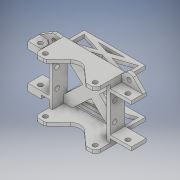
# Autodesk Inventor part: 14HM08 Chassis Flat Bottom
Saved by Autodesk Inventor 2019 (Build 230136000, 136)
## iProperties
Created: 2019-01-31
Part Number: 14HM08 Chassis Flat Bottom
Material: Generic
Document SubType Name: Modeling
Designer: Billy
Density: 1 g/cm^3
Appearance: Red
Author: Billy
Autodesk Inventor part; units mm, degrees
note: some values were not read from the file. Chosen so that the rebuilt part matches the saved one: sketch regions of "Extrusion3".
ref_plane "YZ Plane" through (0, 0, 0) normal (1, 0, 0) x (0, 1, 0)
ref_plane "XZ Plane" through (0, 0, 0) normal (0, 1, 0) x (-1, 0, 0)
sketch "Sketch1" plane through (0, 0, 0) normal (0, 1, 0) x (-1, 0, 0)
  circle A0 centre (21.95, 0) radius 2
  circle A1 centre (-21.95, 0) radius 2
  arc A2 (26.95, 0) -> (18.533144, 3.650355) centre (21.95, 0) ccw
  arc A3 (-18.533144, 3.650355) -> (-26.95, 0) centre (-21.95, 0) ccw
  arc A4 (-6.833713, -7.30071) -> (6.833713, -7.30071) centre (0, 0) ccw
  line L0 (6.833713, -7.30071) -> (18.533144, 3.650355)
  line L1 (-6.833713, -7.30071) -> (-18.533144, 3.650355)
  line L2 (-26.95, 0) -> (-26.95, -18.25)
  line L3 (-26.95, -18.25) -> (26.95, -18.25)
  line L4 (26.95, -18.25) -> (26.95, 0)
  constraints: 10 end point, 6 point on circle, 5 centre point, 4 tangent, 3 coincident, 1 parallel, 5 other
extrude "Extrusion1" add sketch "Sketch1" along normal blind 3
ref_plane "Work Plane1" through (0, 48, 0) normal (0, 1, 0) x (1, 0, 0)
sketch "Sketch2" plane through (0, 48, 0) normal (0, 1, 0) x (1, 0, 0)
  circle A0 centre (21.95, 0) radius 2
  circle A1 centre (-21.95, 0) radius 2
  line L0 (-18.533144, -3.650355) -> (-6.833713, 7.30071)
  arc A2 (6.833713, 7.30071) -> (-6.833713, 7.30071) centre (0, 0) ccw
  line L1 (6.833713, 7.30071) -> (18.533144, -3.650355)
  arc A3 (18.533144, -3.650355) -> (26.95, 0) centre (21.95, 0) ccw
  line L2 (26.95, 0) -> (26.95, 18.25)
  line L3 (26.95, 18.25) -> (-26.95, 18.25)
  line L4 (-26.95, 18.25) -> (-26.95, 0)
  arc A4 (-26.95, 0) -> (-18.533144, -3.650355) centre (-21.95, 0) ccw
extrude "Extrusion2" add sketch "Sketch2" along normal blind 3
sketch "Sketch3" plane through (26.95, 48, -18.25) normal (0, 0, -1) x (-1, 0, 0)
  line L0 (0, 0) -> (53.9, 0)
  line L1 (53.9, 0) -> (53.9, 3)
  line L2 (0, 3) -> (53.9, 3)
  line L3 (0, 0) -> (0, 3)
  line L4 (53.9, -48) -> (0, -48)
  line L5 (53.9, -48) -> (53.9, -45)
  line L6 (0, -45) -> (53.9, -45)
  line L7 (0, -48) -> (0, -45)
  circle A0 centre (-6.625, -46.63) radius 2
  circle A1 centre (-6.625, 1.63) radius 2
  circle A2 centre (59.415, -43.455) radius 2
  circle A3 centre (59.415, -1.545) radius 2
  arc A4 (58.987392, -48.436682) -> (59.415, -38.455) centre (59.415, -43.455) ccw
  arc A5 (-6.625, -41.63) -> (-3.688232, -50.676652) centre (-6.625, -46.63) ccw
  arc A6 (59.415, -6.545) -> (58.987392, 3.436682) centre (59.415, -1.545) ccw
  arc A7 (-3.688232, 5.676652) -> (-6.625, -3.37) centre (-6.625, 1.63) ccw
  line L8 (53.9, -48) -> (0, -48)
  line L9 (0, 3) -> (53.9, 3)
  line L10 (0, -48) -> (-3.688232, -50.676652)
  line L11 (-6.625, -41.63) -> (0, -41.63)
  line L12 (53.9, -48) -> (58.987392, -48.436682)
  line L13 (59.415, -38.455) -> (53.9, -38.455)
  line L14 (53.9, -45) -> (53.9, -48)
  line L15 (0, -48) -> (0, -45)
  line L16 (59.415, -6.545) -> (53.9, -6.545)
  line L17 (53.9, 3) -> (58.987392, 3.436682)
  line L18 (53.9, 3) -> (53.9, 0)
  line L19 (53.9, -6.545) -> (53.9, -38.455)
  line L20 (0, 3) -> (-3.688232, 5.676652)
  line L21 (-6.625, -3.37) -> (0, -3.37)
  line L22 (0, -41.63) -> (0, -3.37)
  line L23 (0, 0) -> (0, 3)
  point P0 (26.95, -48)
  constraints: 36 end point, 10 parallel, 10 perpendicular, 8 centre point, 8 point on circle, 6 tangent, 4 coincident, 2 horizontal, 2 vertical, 8 other
extrude "Extrusion3" add sketch "Sketch3" along normal blind 3
sketch "Sketch4" plane through (26.95, 0, 0) normal (1, 0, 0) x (0, 0, -1)
  line L0 (18.25, 3) -> (0, 3)
  line L1 (7.30071, 48) -> (10, 48)
  line L2 (18.25, 3) -> (8.25, 3)
  line L3 (8.25, 3) -> (8.25, 48)
  line L4 (8.25, 48) -> (18.25, 48)
  line L5 (18.25, 48) -> (18.25, 3)
  point P0 (0, 0)
  dimension "d34" = 10
  constraints: 8 end point, 2 parallel, 1 horizontal, 1 perpendicular, 1 point on line
  measures "d34" distance of L3.end L4.end
extrude "Extrusion4" add sketch "Sketch4" against normal blind 3
sketch "Sketch5" plane through (-26.95, 0, 0) normal (-1, 0, 0) x (0, 0, 1)
  line L0 (-8.25, 3) -> (-18.25, 3) projected
  line L1 (-8.25, 3) -> (-8.25, 48) projected
  line L2 (-18.25, 48) -> (-8.25, 48) projected
  line L3 (-18.25, 3) -> (-18.25, 48) projected
  point P0 (0, 0)
extrude "Extrusion5" add sketch "Sketch5" against normal blind 3
sketch "Sketch6" plane through (26.95, 48, -18.25) normal (0, 0, 1) x (1, 0, 0)
  line L0 (-50.9, -6.860357) -> (-50.9, -38.139643)
  line L1 (-10.302469, -45) -> (-43.597531, -45)
  line L2 (-3, -38.139643) -> (-3, -6.860357)
  line L3 (-10.302469, 0) -> (-43.597531, 0)
  line L4 (-50.9, -38.139643) -> (-34.252469, -22.5)
  line L5 (-26.95, -15.639643) -> (-10.302469, 0)
  line L6 (-10.302469, -45) -> (-26.95, -29.360357)
  line L7 (-34.252469, -22.5) -> (-50.9, -6.860357)
  line L8 (-3, -38.139643) -> (-19.647531, -22.5)
  line L9 (-26.95, -15.639643) -> (-43.597531, 0)
  line L10 (-43.597531, -45) -> (-26.95, -29.360357)
  line L11 (-19.647531, -22.5) -> (-3, -6.860357)
  point P0 (-26.95, -48)
  constraints: 24 end point
extrude "Extrusion6" cut sketch "Sketch6" against normal blind 3
sketch "Sketch8" plane through (26.95, 48, -21.25) normal (0, 0, -1) x (-1, 0, 0)
  line L0 (10.302469, -45) -> (26.95, -29.360357)
  line L1 (26.95, -29.360357) -> (43.597531, -45)
  line L2 (43.597531, -45) -> (10.302469, -45)
  line L3 (43.597531, 0) -> (26.95, -15.639643)
  line L4 (26.95, -15.639643) -> (10.302469, 0)
  line L5 (10.302469, 0) -> (43.597531, 0)
  line L6 (3, -6.860357) -> (19.647531, -22.5)
  line L7 (19.647531, -22.5) -> (3, -38.139643)
  line L8 (3, -38.139643) -> (3, -6.860357)
  line L9 (50.9, -38.139643) -> (34.252469, -22.5)
  line L10 (34.252469, -22.5) -> (50.9, -6.860357)
  line L11 (50.9, -6.860357) -> (50.9, -38.139643)
  circle A0 centre (59.415, -1.545) radius 2
  circle A1 centre (59.415, -43.455) radius 2
  circle A2 centre (-6.625, 1.63) radius 2
  circle A3 centre (-6.625, -46.63) radius 2
  line L12 (0, 3) -> (-3.688232, 5.676652)
  arc A4 (-3.688232, 5.676652) -> (-6.625, -3.37) centre (-6.625, 1.63) ccw
  arc A5 (-6.625, -41.63) -> (-3.688232, -50.676652) centre (-6.625, -46.63) ccw
  line L13 (-3.688232, -50.676652) -> (0, -48)
  line L14 (0, -48) -> (53.9, -48)
  line L15 (53.9, -48) -> (58.987392, -48.436682)
  arc A6 (58.987392, -48.436682) -> (59.415, -38.455) centre (59.415, -43.455) ccw
  line L16 (59.415, -38.455) -> (53.9, -38.455)
  line L17 (57.121975, -6.545) -> (59.415, -6.545)
  arc A7 (59.415, -6.545) -> (58.987392, 3.436682) centre (59.415, -1.545) ccw
  line L18 (58.987392, 3.436682) -> (53.9, 3)
  line L19 (53.9, 3) -> (0, 3)
  line L20 (53.9, -40.75) -> (0, -40.75)
  line L21 (53.9, -4.25) -> (0, -4.25)
  line L22 (0, -41.63) -> (0, -43.75)
  line L23 (0, -1.25) -> (0, -4.25)
  line L24 (0, -40.75) -> (0, -41.63)
  line L25 (63.620113, -43.75) -> (57.436876, -43.75)
  line L26 (53.9, -43.75) -> (0, -43.75)
  line L27 (63.620113, -1.25) -> (57.436876, -1.25)
  line L28 (53.9, -1.25) -> (0, -1.25)
  line L29 (53.9, -43.75) -> (53.9, -40.75)
  line L30 (53.9, -4.25) -> (53.9, -1.25)
  point P0 (26.95, -48)
  constraints: 62 end point, 8 centre point, 4 point on circle, 1 point on line, 18 other
extrude "Extrusion7" add sketch "Sketch8" along normal blind 18 contours L26 L22 L24 L20 L0 | L0 L20 L1 L26 | L1 L20 L29 L26 | L28 L30 L21 L3 | L3 L21 L4 L28 | L4 L21 L23 L28
sketch "Sketch9" plane through (-12.123642, 43.75, -21.25) normal (0, -1, 0) x (1, 0, 0)
  line L0 (24.247285, 0) -> (39.073642, 0)
  line L1 (24.247285, 0) -> (0, 0)
  line L2 (-14.826358, 0) -> (0, 0)
  line L3 (-14.826358, 0) -> (-14.826358, -18)
  line L4 (39.073642, -18) -> (-14.826358, -18)
  line L5 (39.073642, 0) -> (39.073642, -18)
  line L6 (-11.826358, -15) -> (-11.826358, -3)
  line L7 (0, -3) -> (24.247285, -3)
  line L8 (36.073642, -3) -> (36.073642, -15)
  line L9 (23.776294, -15) -> (0.470991, -15)
  line L10 (-8.512342, -18) -> (-14.192846, -19.897014)
  line L11 (38.440131, -19.897014) -> (32.759627, -18)
  line L12 (12.123642, -11.108577) -> (0.470991, -15)
  line L13 (23.776294, -15) -> (12.123642, -11.108577)
  line L14 (5.809627, -9) -> (-11.826358, -14.889568)
  line L15 (-14.826358, -15.891423) -> (-15.459869, -16.102986)
  line L16 (5.809627, -9) -> (-11.826358, -3.110432)
  line L17 (-14.826358, -2.108577) -> (-15.459869, -1.897014)
  line L18 (38.440131, 1.897014) -> (32.759627, 0)
  line L19 (23.776294, -3) -> (12.123642, -6.891423)
  line L20 (-8.512342, 0) -> (-14.192846, 1.897014)
  line L21 (12.123642, -6.891423) -> (0.470991, -3)
  line L22 (39.707154, -16.102986) -> (39.073642, -15.891423)
  line L23 (36.073642, -14.889568) -> (18.437658, -9)
  line L24 (39.707154, -1.897014) -> (39.073642, -2.108577)
  line L25 (36.073642, -3.110432) -> (18.437658, -9)
  point P0 (12.123642, 21.25)
  dimension "d62" = 3
  constraints: 52 end point, 14 point on line
  measures "d62" distance between parallel lines of L4 L9
extrude "Extrusion8" cut sketch "Sketch9" along normal blind 180 and the other way blind 9 contours L6 L16 L14 | L7 L19 L21 | L8 L23 L25 | L9 L12 L13
sketch "Sketch13" plane through (26.95, 48, -21.25) normal (0, 0, -1) x (-1, 0, 0)
  line L0 (-6.625, -3.37) -> (0, -3.37)
  line L1 (0, -3.37) -> (-6.625, -3.37)
  line L2 (-11.625, 1.63) -> (-11.625, -6.37)
  line L3 (-11.625, -6.37) -> (0, -6.37)
  line L4 (0, -6.37) -> (0, -3.37)
  line L5 (0, -1.25) -> (11.633024, -1.25)
  line L6 (11.633024, -1.25) -> (10.302469, 0)
  line L7 (10.302469, 0) -> (43.597531, 0)
  line L8 (43.597531, 0) -> (42.266976, -1.25)
  line L9 (42.266976, -1.25) -> (53.9, -1.25)
  line L10 (53.9, -1.25) -> (53.9, -4.25)
  line L11 (53.9, -4.25) -> (39.073642, -4.25)
  line L12 (39.073642, -4.25) -> (26.95, -15.639643)
  line L13 (26.95, -15.639643) -> (14.826358, -4.25)
  line L14 (14.826358, -4.25) -> (0, -4.25)
  line L15 (0, -4.25) -> (0, -40.75)
  line L16 (0, -40.75) -> (14.826358, -40.75)
  line L17 (14.826358, -40.75) -> (26.95, -29.360357)
  line L18 (26.95, -29.360357) -> (39.073642, -40.75)
  line L19 (39.073642, -40.75) -> (53.9, -40.75)
  line L20 (53.9, -40.75) -> (53.9, -43.75)
  line L21 (53.9, -43.75) -> (42.266976, -43.75)
  line L22 (42.266976, -43.75) -> (43.597531, -45)
  line L23 (43.597531, -45) -> (10.302469, -45)
  line L24 (10.302469, -45) -> (11.633024, -43.75)
  line L25 (11.633024, -43.75) -> (0, -43.75)
  line L26 (0, -43.75) -> (0, -43.373437)
  line L27 (0, -41.63) -> (-6.625, -41.63)
  arc A0 (-6.625, -41.63) -> (-11.625, -46.63) centre (-6.625, -46.63) ccw
  line L28 (-3.688232, -50.676652) -> (0, -48)
  line L29 (0, -48) -> (53.9, -48)
  line L30 (53.9, -48) -> (58.987392, -48.436682)
  arc A1 (58.987392, -48.436682) -> (59.415, -38.455) centre (59.415, -43.455) ccw
  line L31 (59.415, -38.455) -> (53.9, -38.455)
  line L32 (53.9, -38.455) -> (53.9, -6.545)
  line L33 (53.9, -6.545) -> (59.415, -6.545)
  arc A2 (59.415, -6.545) -> (58.987392, 3.436682) centre (59.415, -1.545) ccw
  line L34 (58.987392, 3.436682) -> (53.9, 3)
  line L35 (53.9, 3) -> (0, 3)
  line L36 (0, 3) -> (-3.688232, 5.676652)
  arc A3 (-11.625, 1.63) -> (-6.625, -3.37) centre (-6.625, 1.63) ccw
  line L37 (-6.625, -3.37) -> (0, -3.37)
  line L38 (0, -3.37) -> (0, -1.25)
  line L39 (3, -6.860357) -> (19.647531, -22.5)
  line L40 (19.647531, -22.5) -> (3, -38.139643)
  line L41 (3, -38.139643) -> (3, -6.860357)
  line L42 (50.9, -38.139643) -> (34.252469, -22.5)
  line L43 (34.252469, -22.5) -> (50.9, -6.860357)
  line L44 (50.9, -6.860357) -> (50.9, -38.139643)
  circle A4 centre (59.415, -1.545) radius 2
  circle A5 centre (59.415, -43.455) radius 2
  circle A6 centre (-6.625, 1.63) radius 2
  circle A7 centre (-6.625, -46.63) radius 2
  line L45 (0, -41.63) -> (-6.625, -41.63)
  line L46 (-11.625, -46.63) -> (-11.625, -38.63)
  line L47 (-11.625, -38.63) -> (0, -38.63)
  line L48 (0, -38.63) -> (0, -41.63)
  point P0 (26.95, -48)
  constraints: 30 end point, 12 centre point, 4 point on circle, 1 point on line
extrude "Extrusion11" add sketch "Sketch13" against normal up to surface (3 mm away) contours L0 L4 L3 L2 A3 | L15 L48 L27 A0 L46 L47
sketch "Sketch14" plane through (26.95, 48, -18.25) normal (0, 0, 1) x (1, 0, 0)
  line L0 (0, -48) -> (0, -38.63)
  line L1 (3.688232, -50.676652) -> (0, -48)
  arc A0 (3.688232, -50.676652) -> (11.625, -46.63) centre (6.625, -46.63) ccw
  line L2 (11.625, -38.63) -> (11.625, -46.63)
  line L3 (0, -38.63) -> (11.625, -38.63)
  circle A1 centre (6.625, -46.63) radius 2
  circle A2 centre (6.625, 1.63) radius 2
  line L4 (0, -6.37) -> (0, 3)
  line L5 (11.625, -6.37) -> (0, -6.37)
  line L6 (11.625, 1.63) -> (11.625, -6.37)
  arc A3 (11.625, 1.63) -> (3.688232, 5.676652) centre (6.625, 1.63) ccw
  line L7 (0, 3) -> (3.688232, 5.676652)
  line L8 (0, -1.25) -> (0, -4.25)
  line L9 (11.625, -6.37) -> (0, -6.37)
  line L10 (0, -6.37) -> (0, -3.37)
  line L11 (0, -3.37) -> (11.625, -3.37)
  line L12 (11.625, -3.37) -> (11.625, -6.37)
  line L13 (11.625, -38.63) -> (0, -38.63)
  line L14 (0, -38.63) -> (0, -41.63)
  line L15 (0, -41.63) -> (11.625, -41.63)
  line L16 (11.625, -41.63) -> (11.625, -38.63)
  point P0 (-26.95, -48)
  dimension "d92" = 3
  dimension "d93" = 3
  constraints: 16 end point, 4 parallel, 2 horizontal, 2 perpendicular, 2 point on line
  measures "d92" distance of L9.end L10.end
  measures "d93" distance of L14.end L13.end
extrude "Extrusion12" add sketch "Sketch14" along normal blind 10 contours L0 L3 L2 L15 | L4 L11 L6 L5
sketch "Sketch15" plane through (38.575, 41.63, -21.25) normal (1, 0, 0) x (0, 0, -1)
  line L0 (-3, -35.26) -> (-3, -40.26) projected
  line L1 (-3, -40.26) -> (0, -40.26) projected
  line L2 (0, -32.26) -> (0, -40.26) projected
  line L3 (0, -32.26) -> (-13, -32.26) projected
  line L4 (-13, -35.26) -> (-13, -32.26) projected
  line L5 (-3, -35.26) -> (-13, -35.26) projected
  line L6 (-3, 8) -> (-3, 3) projected
  line L7 (-3, 3) -> (-13, 3) projected
  line L8 (-13, 0) -> (-13, 3) projected
  line L9 (0, 0) -> (-13, 0) projected
  line L10 (0, 8) -> (0, 0) projected
  line L11 (-3, 8) -> (0, 8) projected
  line L12 (0, -32.26) -> (-13, -32.26) projected
  line L13 (-13, -35.26) -> (0, -35.26)
  line L14 (0, -35.26) -> (0, -32.26)
  line L15 (0, -32.26) -> (-13, -32.26)
  line L16 (-13, -32.26) -> (-13, -35.26)
  line L17 (-13, 0) -> (0, 0)
  line L18 (0, 0) -> (0, 3)
  line L19 (0, 3) -> (-13, 3)
  line L20 (-13, 3) -> (-13, 0)
  point P0 (-21.25, -41.63)
  constraints: 16 end point, 4 parallel, 2 horizontal, 2 perpendicular, 1 point on line
extrude "Extrusion13" add sketch "Sketch15" along normal blind 7 contours L5 L4 L3 L2 L13 | L19 L10 L9 L8 L7
sketch "Sketch16" plane through (26.95, 44.63, -18.25) normal (0, 1, 0) x (1, 0, 0)
  line L0 (0, 0) -> (11.625, 0) projected
  line L1 (0, -10) -> (0, 0) projected
  line L2 (0, -10) -> (18.625, -10) projected
  line L3 (18.625, 3) -> (18.625, -10) projected
  line L4 (11.625, 3) -> (18.625, 3) projected
  line L5 (11.625, 0) -> (11.625, 3) projected
  line L6 (18.625, -10) -> (11.625, -10)
  line L7 (11.625, -6) -> (18.625, -6)
  line L8 (18.625, -6) -> (18.625, -10)
  circle A0 centre (11.625, -6) radius 2
  point P0 (-26.95, -18.25)
  dimension "d98" = 7
  dimension "d99" = 4
  dimension "d100" = 4
  constraints: 6 end point, 1 centre point, 1 coincident, 1 horizontal, 1 parallel
  measures "d98" distance of L7.start L7.end
  measures "d99" distance of L6.end L7.start
  measures "d100" diameter of A0
extrude "Extrusion14" cut sketch "Sketch16" along normal blind 100 and the other way blind 200 contours A0
sketch "Sketch17" plane through (26.95, 48, -18.25) normal (0, 0, 1) x (1, 0, 0)
  circle A0 centre (-59.415, -1.545) radius 2
  line L0 (-58.987392, 3.436682) -> (-53.9, 3)
  arc A1 (-64.410418, -1.759) -> (-59.415, -6.545) centre (-59.415, -1.545) ccw
  line L1 (-53.9, -6.545) -> (-59.415, -6.545)
  line L2 (-59.415, -38.455) -> (-53.9, -38.455)
  arc A2 (-59.415, -38.455) -> (-64.410418, -43.241) centre (-59.415, -43.455) ccw
  line L3 (-53.9, -48) -> (-58.987392, -48.436682)
  circle A3 centre (-59.415, -43.455) radius 2
  line L4 (-53.9, -6.545) -> (-59.415, -6.545)
  line L5 (-64.410418, -1.759) -> (-64.410418, -9.545)
  line L6 (-64.410418, -9.545) -> (-53.9, -9.545)
  line L7 (-53.9, -9.545) -> (-53.9, -6.545)
  line L8 (-53.9, -38.455) -> (-59.415, -38.455)
  line L9 (-64.410418, -43.241) -> (-64.410418, -35.455)
  line L10 (-64.410418, -35.455) -> (-53.9, -35.455)
  line L11 (-53.9, -35.455) -> (-53.9, -38.455)
  point P0 (-26.95, -48)
  constraints: 24 end point, 8 centre point, 4 point on circle
extrude "Extrusion15" add sketch "Sketch17" against normal up to surface (3 mm away) contours A1 L1 L7 L6 L5 | A2 L9 L10 L11 L2
sketch "Sketch19" plane through (26.95, 48, -18.25) normal (0, 0, 1) x (1, 0, 0)
  circle A0 centre (-59.415, -1.545) radius 2
  line L0 (-53.9, 3) -> (-53.9, -9.545)
  line L1 (-58.987392, 3.436682) -> (-53.9, 3)
  arc A1 (-58.987392, 3.436682) -> (-64.410418, -1.759) centre (-59.415, -1.545) ccw
  line L2 (-64.410418, -1.759) -> (-64.410418, -9.545)
  line L3 (-64.410418, -9.545) -> (-53.9, -9.545)
  line L4 (-53.9, -35.455) -> (-53.9, -48)
  line L5 (-53.9, -35.455) -> (-64.410418, -35.455)
  line L6 (-64.410418, -35.455) -> (-64.410418, -43.241)
  arc A2 (-64.410418, -43.241) -> (-58.987392, -48.436682) centre (-59.415, -43.455) ccw
  line L7 (-53.9, -48) -> (-58.987392, -48.436682)
  circle A3 centre (-59.415, -43.455) radius 2
  line L8 (-64.410418, -9.545) -> (-53.9, -9.545)
  line L9 (-64.410418, -9.545) -> (-53.9, -9.545)
  line L10 (-53.9, -9.545) -> (-53.9, -6.545)
  line L11 (-53.9, -6.545) -> (-64.410418, -6.545)
  line L12 (-64.410418, -6.545) -> (-64.410418, -9.545)
  line L13 (-53.9, -45) -> (-53.9, 0)
  line L14 (-64.410418, -35.455) -> (-53.9, -35.455)
  line L15 (-53.9, -35.455) -> (-53.9, -38.455)
  line L16 (-53.9, -38.455) -> (-64.410418, -38.455)
  line L17 (-64.410418, -38.455) -> (-64.410418, -35.455)
  point P0 (-26.95, -48)
  dimension "d110" = 3
  dimension "d111" = 3
  constraints: 16 end point, 4 parallel, 2 horizontal, 2 perpendicular, 2 point on line
  measures "d110" distance of L10.end L9.end
  measures "d111" distance of L14.end L15.end
extrude "Extrusion16" add sketch "Sketch19" along normal up to surface (10 mm away) contours L0 L3 L2 L11 | L4 L16 L6 L5
sketch "Sketch20" plane through (-37.460418, 38.455, -21.25) normal (-1, 0, 0) x (0, 0, 1)
  line L0 (0, 7.786) -> (0, 0) projected
  line L1 (0, 0) -> (13, 0) projected
  line L2 (13, 0) -> (13, 3) projected
  line L3 (3, 3) -> (13, 3) projected
  line L4 (3, 7.786) -> (3, 3) projected
  line L5 (0, 7.786) -> (3, 7.786) projected
  line L6 (0, -25.91) -> (0, -33.696) projected
  line L7 (3, -33.696) -> (0, -33.696) projected
  line L8 (3, -28.91) -> (3, -33.696) projected
  line L9 (3, -28.91) -> (13, -28.91) projected
  line L10 (13, -28.91) -> (13, -25.91) projected
  line L11 (0, -25.91) -> (13, -25.91) projected
  line L12 (13, 3) -> (0, 3)
  line L13 (0, 3) -> (0, 0)
  line L14 (0, 0) -> (13, 0)
  line L15 (13, 0) -> (13, 3)
  line L16 (13, -28.91) -> (13, -25.91) projected
  line L17 (0, -25.91) -> (13, -25.91)
  line L18 (13, -25.91) -> (13, -28.91)
  line L19 (13, -28.91) -> (0, -28.91)
  line L20 (0, -28.91) -> (0, -25.91)
  point P0 (21.25, -38.455)
  constraints: 16 end point, 4 parallel, 2 horizontal, 2 perpendicular
extrude "Extrusion17" add sketch "Sketch20" along normal blind 8.115 contours L12 L3 L2 L1 L0 | L11 L10 L9 L19 L6
sketch "Sketch21" plane through (-37.460418, 41.455, -18.25) normal (0, 1, 0) x (1, 0, 0)
  line L0 (10.510418, -10) -> (-8.115, -10)
  line L1 (-8.115, -10) -> (-1.115, -10)
  line L2 (-1.115, -6) -> (-8.115, -6)
  line L3 (-8.115, -6) -> (-8.115, -10)
  circle A0 centre (-1.115, -6) radius 2
  point P0 (37.460418, -18.25)
  dimension "d116" = 7
  dimension "d117" = 4
  dimension "d118" = 4
  constraints: 6 end point, 1 centre point, 1 coincident, 1 horizontal, 1 parallel
  measures "d116" distance of L2.end L2.start
  measures "d117" distance of L2.start L1.end
  measures "d118" diameter of A0
extrude "Extrusion18" cut sketch "Sketch21" against normal blind 50.49
sketch "Sketch22" plane through (-37.460418, 41.455, -18.25) normal (0, 1, 0) x (1, 0, 0)
  circle A0 centre (-1.115, -6) radius 2
  arc A1 (3.885, -6) -> (0, -1.125908) centre (-1.115, -6) ccw
  circle A2 centre (-1.115, -6) radius 2
  line L0 (10.510418, -10) -> (-8.115, -10)
  line L1 (10.510418, 0) -> (10.510418, -10)
  line L2 (0, 0) -> (10.510418, 0)
  line L3 (0, 3) -> (0, 0)
  line L4 (0, 3) -> (-8.115, 3)
  line L5 (-8.115, -10) -> (-8.115, 3)
  line L6 (3.885, -6) -> (3.885, -10)
  line L7 (0, 0) -> (0, -1.125908)
  point P0 (37.460418, -18.25)
  dimension "d121" = 10
  constraints: 4 end point, 2 point on circle, 2 vertical, 1 centre point, 1 coincident, 1 point on line
  measures "d121" diameter of A1
extrude "Extrusion19" add sketch "Sketch22" along normal blind 3.175 contours L6 L0 L5 L4 L3 L7 A1
sketch "Sketch23" plane through (-37.460418, 9.545, -18.25) normal (0, -1, 0) x (1, 0, 0)
  circle A0 centre (-1.115, 6) radius 2
  line L0 (-8.115, 10) -> (3.885, 10)
  line L1 (3.885, 10) -> (3.885, 6)
  arc A1 (0, 1.125908) -> (3.885, 6) centre (-1.115, 6) ccw
  line L2 (0, 1.125908) -> (0, 0)
  line L3 (0, -3) -> (0, 0)
  line L4 (0, -3) -> (-8.115, -3)
  line L5 (-8.115, -3) -> (-8.115, 10)
  point P0 (37.460418, 18.25)
extrude "Extrusion20" add sketch "Sketch23" along normal blind 3.175
sketch "Sketch24" plane through (26.95, 48, -21.25) normal (0, 0, -1) x (-1, 0, 0)
  line L0 (0, -6.37) -> (0, -38.63)
  line L1 (0, -38.63) -> (-18.625, -38.63)
  line L2 (-18.625, -41.63) -> (-18.625, -38.63)
  line L3 (-11.625, -41.63) -> (-18.625, -41.63)
  line L4 (-11.625, -41.63) -> (-11.625, -46.63)
  arc A0 (-11.625, -46.63) -> (-3.688232, -50.676652) centre (-6.625, -46.63) ccw
  line L5 (-3.688232, -50.676652) -> (0, -48)
  line L6 (0, -48) -> (53.9, -48)
  line L7 (53.9, -48) -> (58.987392, -48.436682)
  arc A1 (58.987392, -48.436682) -> (64.410418, -43.241) centre (59.415, -43.455) ccw
  line L8 (64.410418, -40.955) -> (64.410418, -43.241)
  line L9 (72.525418, -40.955) -> (64.410418, -40.955)
  line L10 (72.525418, -35.455) -> (72.525418, -40.955)
  line L11 (53.9, -35.455) -> (72.525418, -35.455)
  line L12 (53.9, -35.455) -> (53.9, -9.545)
  line L13 (53.9, -9.545) -> (72.525418, -9.545)
  line L14 (72.525418, -9.545) -> (72.525418, -4.045)
  line L15 (64.410418, -4.045) -> (72.525418, -4.045)
  line L16 (64.410418, -1.759) -> (64.410418, -4.045)
  arc A2 (64.410418, -1.759) -> (58.987392, 3.436682) centre (59.415, -1.545) ccw
  line L17 (58.987392, 3.436682) -> (53.9, 3)
  line L18 (53.9, 3) -> (0, 3)
  line L19 (0, 3) -> (-3.688232, 5.676652)
  arc A3 (-3.688232, 5.676652) -> (-11.625, 1.63) centre (-6.625, 1.63) ccw
  line L20 (-11.625, 1.63) -> (-11.625, -3.37)
  line L21 (-11.625, -3.37) -> (-18.625, -3.37)
  line L22 (-18.625, -6.37) -> (-18.625, -3.37)
  line L23 (-18.625, -6.37) -> (0, -6.37)
  line L24 (0, -1.25) -> (0, -4.25)
  line L25 (0, -1.25) -> (11.633024, -1.25)
  line L26 (11.633024, -1.25) -> (10.302469, 0)
  line L27 (10.302469, 0) -> (43.597531, 0)
  line L28 (43.597531, 0) -> (42.266976, -1.25)
  line L29 (42.266976, -1.25) -> (53.9, -1.25)
  line L30 (53.9, -1.25) -> (53.9, -4.25)
  line L31 (53.9, -4.25) -> (39.073642, -4.25)
  line L32 (39.073642, -4.25) -> (26.95, -15.639643)
  line L33 (26.95, -15.639643) -> (14.826358, -4.25)
  line L34 (14.826358, -4.25) -> (0, -4.25)
  line L35 (0, -40.75) -> (0, -43.75)
  line L36 (0, -40.75) -> (14.826358, -40.75)
  line L37 (14.826358, -40.75) -> (26.95, -29.360357)
  line L38 (26.95, -29.360357) -> (39.073642, -40.75)
  line L39 (39.073642, -40.75) -> (53.9, -40.75)
  line L40 (53.9, -40.75) -> (53.9, -43.75)
  line L41 (53.9, -43.75) -> (42.266976, -43.75)
  line L42 (42.266976, -43.75) -> (43.597531, -45)
  line L43 (43.597531, -45) -> (10.302469, -45)
  line L44 (10.302469, -45) -> (11.633024, -43.75)
  line L45 (11.633024, -43.75) -> (0, -43.75)
  line L46 (3, -6.860357) -> (19.647531, -22.5)
  line L47 (19.647531, -22.5) -> (3, -38.139643)
  line L48 (3, -38.139643) -> (3, -6.860357)
  line L49 (50.9, -38.139643) -> (34.252469, -22.5)
  line L50 (34.252469, -22.5) -> (50.9, -6.860357)
  line L51 (50.9, -6.860357) -> (50.9, -38.139643)
  circle A4 centre (59.415, -1.545) radius 2
  circle A5 centre (59.415, -43.455) radius 2
  circle A6 centre (-6.625, 1.63) radius 2
  circle A7 centre (-6.625, -46.63) radius 2
  line L52 (-18.625, -3.37) -> (-10.175296, 5.15071)
  arc A8 (-3.688232, 5.676652) -> (-11.625, 1.63) centre (-6.625, 1.63) ccw
  line L53 (-18.625, -41.63) -> (-10.175296, -50.15071)
  line L54 (72.525418, -4.045) -> (62.123336, 2.657965)
  line L55 (72.525418, -40.955) -> (62.123336, -47.657965)
  point P0 (26.95, -48)
  point P1 (64.410418, -2.902)
  constraints: 112 end point, 16 centre point, 12 point on circle, 6 vertical, 4 horizontal, 4 tangent, 1 midpoint, 6 other
extrude "Extrusion21" add sketch "Sketch24" against normal up to surface (3 mm away) contours L52 A3 L20 L21 | L3 L4 A0 L53 | L54 L15 L16 A2 | A1 L8 L9 L55
sketch "Sketch25" plane through (26.95, 9.37, -8.25) normal (1, 0, 0) x (0, 0, -1)
  line L0 (0, 0) -> (13, 0) projected
  line L1 (13, 32.26) -> (13, 0) projected
  line L2 (13, 32.26) -> (0, 32.26) projected
  line L3 (0, 0) -> (0, 32.26) projected
  line L4 (13, 32.26) -> (0, 32.26) projected
  line L5 (0, 32.26) -> (4, 32.26)
  line L6 (4, 32.26) -> (4, 24.26)
  line L7 (4, 24.26) -> (0, 24.26)
  line L8 (0, 24.26) -> (0, 32.26)
  line L9 (0, 0) -> (4, 0)
  line L10 (4, 0) -> (4, 8)
  line L11 (4, 8) -> (0, 8)
  line L12 (0, 8) -> (0, 0)
  circle A0 centre (4, 24.26) radius 2
  circle A1 centre (4, 8) radius 2
  point P0 (-8.25, -9.37)
  dimension "d128" = 4
  dimension "d129" = 8
  dimension "d130" = 4
  dimension "d131" = 8
  dimension "d132" = 4
  dimension "d133" = 4
  constraints: 16 end point, 4 parallel, 2 centre point, 2 coincident, 2 horizontal, 2 perpendicular
  measures "d128" distance of L6.end L7.end
  measures "d129" distance of L5.end L6.end
  measures "d130" distance of L11.end L10.end
  measures "d131" distance of L10.end L9.end
  measures "d132" diameter of A0
  measures "d133" diameter of A1
extrude "Extrusion22" cut sketch "Sketch25" against normal blind 4 contours A1 L11 L10 | L10 L11 A1 | A0 L6 L7 | L7 L6 A0
sketch "Sketch27" plane through (-26.95, 12.545, -8.25) normal (-1, 0, 0) x (0, 0, 1)
  circle A0 centre (-4, 4.825) radius 2
  circle A1 centre (-4, 21.085) radius 2
  line L0 (0, -9.545) -> (-10, -9.545)
  line L1 (0, -9.545) -> (0, 35.455)
  line L2 (-10, 35.455) -> (0, 35.455)
  line L3 (-10, 28.594643) -> (-10, 35.455)
  line L4 (-10, 28.594643) -> (-13, 28.594643)
  line L5 (-13, -2.684643) -> (-13, 28.594643)
  line L6 (-10, -2.684643) -> (-13, -2.684643)
  line L7 (-10, -9.545) -> (-10, -2.684643)
  point P0 (8.25, -12.545)
extrude "Extrusion23" cut sketch "Sketch27" against normal blind 4 contours A0 | A1
sketch "Sketch28" plane through (26.95, 48, -21.25) normal (0, 0, -1) x (-1, 0, 0)
  line L0 (0, -1.25) -> (0, -4.25)
  line L1 (0, -1.25) -> (11.633024, -1.25)
  line L2 (11.633024, -1.25) -> (10.302469, 0)
  line L3 (10.302469, 0) -> (43.597531, 0)
  line L4 (43.597531, 0) -> (42.266976, -1.25)
  line L5 (42.266976, -1.25) -> (53.9, -1.25)
  line L6 (53.9, -1.25) -> (53.9, -4.25)
  line L7 (53.9, -4.25) -> (39.073642, -4.25)
  line L8 (39.073642, -4.25) -> (26.95, -15.639643)
  line L9 (26.95, -15.639643) -> (14.826358, -4.25)
  line L10 (14.826358, -4.25) -> (0, -4.25)
  line L11 (0, -40.75) -> (0, -43.75)
  line L12 (0, -40.75) -> (14.826358, -40.75)
  line L13 (14.826358, -40.75) -> (26.95, -29.360357)
  line L14 (26.95, -29.360357) -> (39.073642, -40.75)
  line L15 (39.073642, -40.75) -> (53.9, -40.75)
  line L16 (53.9, -40.75) -> (53.9, -43.75)
  line L17 (53.9, -43.75) -> (42.266976, -43.75)
  line L18 (42.266976, -43.75) -> (43.597531, -45)
  line L19 (43.597531, -45) -> (10.302469, -45)
  line L20 (10.302469, -45) -> (11.633024, -43.75)
  line L21 (11.633024, -43.75) -> (0, -43.75)
  line L22 (3, -6.860357) -> (19.647531, -22.5)
  line L23 (19.647531, -22.5) -> (3, -38.139643)
  line L24 (3, -38.139643) -> (3, -6.860357)
  line L25 (50.9, -38.139643) -> (34.252469, -22.5)
  line L26 (34.252469, -22.5) -> (50.9, -6.860357)
  line L27 (50.9, -6.860357) -> (50.9, -38.139643)
  circle A0 centre (59.415, -1.545) radius 2
  circle A1 centre (59.415, -43.455) radius 2
  circle A2 centre (-6.625, 1.63) radius 2
  circle A3 centre (-6.625, -46.63) radius 2
  line L28 (72.525418, -9.545) -> (72.525418, -3.37)
  line L29 (71.477911, -3.37) -> (72.525418, -3.37)
  line L30 (71.477911, -3.37) -> (62.123336, 2.657965)
  arc A4 (62.123336, 2.657965) -> (58.987392, 3.436682) centre (59.415, -1.545) ccw
  line L31 (58.987392, 3.436682) -> (53.9, 3)
  line L32 (53.9, 3) -> (0, 3)
  line L33 (0, 3) -> (-3.688232, 5.676652)
  arc A5 (-3.688232, 5.676652) -> (-10.175296, 5.15071) centre (-6.625, 1.63) ccw
  line L34 (-10.175296, 5.15071) -> (-18.625, -3.37)
  line L35 (-18.625, -6.37) -> (-18.625, -3.37)
  line L36 (-18.625, -6.37) -> (0, -6.37)
  line L37 (0, -6.37) -> (0, -38.63)
  line L38 (0, -38.63) -> (-18.625, -38.63)
  line L39 (-18.625, -41.63) -> (-18.625, -38.63)
  line L40 (-18.625, -41.63) -> (-10.175296, -50.15071)
  arc A6 (-10.175296, -50.15071) -> (-3.688232, -50.676652) centre (-6.625, -46.63) ccw
  line L41 (-3.688232, -50.676652) -> (0, -48)
  line L42 (0, -48) -> (53.9, -48)
  line L43 (53.9, -48) -> (58.987392, -48.436682)
  arc A7 (58.987392, -48.436682) -> (62.123336, -47.657965) centre (59.415, -43.455) ccw
  line L44 (62.123336, -47.657965) -> (71.477911, -41.63)
  line L45 (72.525418, -41.63) -> (71.477911, -41.63)
  line L46 (72.525418, -35.455) -> (72.525418, -41.63)
  line L47 (53.9, -35.455) -> (72.525418, -35.455)
  line L48 (53.9, -35.455) -> (53.9, -9.545)
  line L49 (53.9, -9.545) -> (72.525418, -9.545)
  line L50 (72.525418, -41.63) -> (61.923925, -47.779962)
  line L51 (72.525418, -3.37) -> (61.923925, 2.779962)
  arc A8 (58.987392, -48.436682) -> (62.123336, -47.657965) centre (59.415, -43.455) ccw
  point P0 (26.95, -48)
  point P1 (64.410418, -38.455)
  point P2 (72.001665, -3.37)
  constraints: 104 end point, 16 centre point, 10 point on circle, 2 tangent, 2 vertical, 1 horizontal, 1 midpoint, 5 other
extrude "Extrusion24" add sketch "Sketch28" against normal up to surface (3 mm away) contours L29 L30 A4 L51 | L50 A7 L44 L45
sketch "Sketch30" plane through (0, 51, 0) normal (0, 1, 0) x (1, 0, 0)
  circle A0 centre (-21.95, 0) radius 2
  circle A1 centre (21.95, 0) radius 2
  arc A2 (6.833713, 7.30071) -> (-6.833713, 7.30071) centre (0, 0) ccw
  line L0 (26.95, 0) -> (26.95, 18.25)
  line L1 (26.95, 18.25) -> (26.95, 21.25)
  line L2 (-26.95, 21.25) -> (26.95, 21.25)
  line L3 (-26.95, 18.25) -> (-26.95, 21.25)
  line L4 (-26.95, 18.25) -> (-26.95, 0)
  line L5 (-6.150342, 6.570639) -> (-17.977518, -4.5)
  line L6 (-27.95, 18.25) -> (-27.95, 22.25)
  line L7 (27.95, 22.25) -> (27.95, 18.25)
  arc A3 (17.849772, -4.380426) -> (17.981373, -4.5) centre (21.95, 0) ccw
  line L8 (17.849772, -4.380426) -> (6.150342, 6.570639)
  arc A4 (6.150342, 6.570639) -> (-6.150342, 6.570639) centre (0, 0) ccw
  arc A5 (-26.95, 0) -> (-24.129449, -4.5) centre (-21.95, 0) ccw
  line L9 (-24.129449, -4.5) -> (-17.977518, -4.5)
  line L10 (17.981373, -4.5) -> (24.129449, -4.5)
  arc A6 (24.129449, -4.5) -> (26.95, 0) centre (21.95, 0) ccw
  constraints: 22 end point, 10 point on circle, 9 centre point
extrude "Extrusion25" add sketch "Sketch30" against normal up to surface (3 mm away)
sketch "Sketch31" plane through (0, 51, 0) normal (0, 1, 0) x (1, 0, 0)
  arc A0 (19.770551, -4.5) -> (24.129449, -4.5) centre (21.95, 0) ccw
  line L0 (26.95, 0) -> (26.95, 18.25)
  line L1 (26.95, 18.25) -> (26.95, 21.25)
  line L2 (-26.95, 21.25) -> (26.95, 21.25)
  line L3 (-26.95, 18.25) -> (-26.95, 21.25)
  line L4 (-26.95, 18.25) -> (-26.95, 0)
  arc A1 (-24.129449, -4.5) -> (-19.770551, -4.5) centre (-21.95, 0) ccw
  line L5 (-24.129449, -4.5) -> (-19.770551, -4.5)
  line L6 (-17.977518, -4.5) -> (-6.150342, 6.570639)
  arc A2 (6.150342, 6.570639) -> (-6.150342, 6.570639) centre (0, 0) ccw
  line L7 (6.150342, 6.570639) -> (17.849772, -4.380426)
  arc A3 (17.849772, -4.380426) -> (17.981373, -4.5) centre (21.95, 0) ccw
  line L8 (19.770551, -4.5) -> (24.129449, -4.5)
  circle A4 centre (21.95, 0) radius 2
  circle A5 centre (-21.95, 0) radius 2
  constraints: 18 end point, 11 centre point, 8 point on circle
extrude "Extrusion26" cut sketch "Sketch31" against normal blind 3 contours L8 A0 | L5 A1
fillet "Fillet2" radius 2 2 edges at (-17.9775, 49.5, 4.5) (17.9814, 49.5, 4.5)
sketch "Sketch32" plane through (0, 0, 0) normal (0, -1, 0) x (1, 0, 0)
  arc A0 (18.76751, 4.5) -> (17.400767, 3.960142) centre (18.76751, 2.5) ccw
  line L0 (6.150342, -6.570639) -> (17.400767, 3.960142)
  arc A1 (-6.150342, -6.570639) -> (6.150342, -6.570639) centre (0, 0) ccw
  line L1 (-17.400767, 3.960142) -> (-6.150342, -6.570639)
  arc A2 (-17.400767, 3.960142) -> (-18.76751, 4.5) centre (-18.76751, 2.5) ccw
  line L2 (-18.76751, 4.5) -> (-24.129449, 4.5)
  arc A3 (-24.129449, 4.5) -> (-26.95, 0) centre (-21.95, 0) ccw
  line L3 (-26.95, -8.25) -> (-26.95, 0)
  line L4 (-26.95, -8.25) -> (-23.95, -8.25)
  line L5 (-23.95, -8.25) -> (-23.95, -18.25)
  line L6 (-16.647531, -18.25) -> (-23.95, -18.25)
  line L7 (-16.647531, -18.25) -> (-16.647531, -21.25)
  line L8 (16.647531, -21.25) -> (-16.647531, -21.25)
  line L9 (16.647531, -18.25) -> (16.647531, -21.25)
  line L10 (23.95, -18.25) -> (16.647531, -18.25)
  line L11 (23.95, -18.25) -> (23.95, -8.25)
  line L12 (23.95, -8.25) -> (26.95, -8.25)
  line L13 (26.95, 0) -> (26.95, -8.25)
  arc A4 (26.95, 0) -> (24.129449, 4.5) centre (21.95, 0) ccw
  line L14 (24.129449, 4.5) -> (18.76751, 4.5)
  circle A5 centre (21.95, 0) radius 2
  circle A6 centre (-21.95, 0) radius 2
extrude "Extrusion27" add sketch "Sketch32" against normal up to surface (3 mm away)
sketch "Sketch33" plane through (0, 0, 0) normal (0, -1, 0) x (1, 0, 0)
  circle A0 centre (21.95, 0) radius 2
  circle A1 centre (-21.95, 0) radius 2
  arc A2 (24.129449, 4.5) -> (19.770551, 4.5) centre (21.95, 0) ccw
  line L0 (24.129449, 4.5) -> (19.770551, 4.5)
  arc A3 (18.76751, 4.5) -> (17.400767, 3.960142) centre (18.76751, 2.5) ccw
  line L1 (17.400767, 3.960142) -> (6.150342, -6.570639)
  arc A4 (-6.150342, -6.570639) -> (6.150342, -6.570639) centre (0, 0) ccw
  line L2 (-6.150342, -6.570639) -> (-17.400767, 3.960142)
  arc A5 (-17.400767, 3.960142) -> (-18.76751, 4.5) centre (-18.76751, 2.5) ccw
  line L3 (-19.770551, 4.5) -> (-24.129449, 4.5)
  arc A6 (-19.770551, 4.5) -> (-24.129449, 4.5) centre (-21.95, 0) ccw
  line L4 (-26.95, 0) -> (-26.95, -18.25)
  line L5 (-26.95, -18.25) -> (-26.95, -21.25)
  line L6 (26.95, -21.25) -> (-26.95, -21.25)
  line L7 (26.95, -18.25) -> (26.95, -21.25)
  line L8 (26.95, -18.25) -> (26.95, 0)
  constraints: 18 end point, 13 centre point, 10 point on circle
extrude "Extrusion28" cut sketch "Sketch33" against normal blind 3 contours L0 A2 | L3 A6
body "Solid1"
